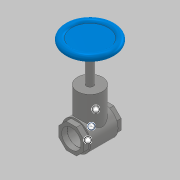
# Autodesk Inventor part: Manual Threaded Ball Valve DN40 S235
Saved by Autodesk Inventor 2017 (Build 210142000, 142)
## iProperties
Created: 2017-11-25
Part Number: Manual Threaded Ball Valve DN40 S235
Material: S235
Document SubType Name: Modeling
Designer: Demarec
Density: 7.85 g/cm^3
Appearance: Plate(1)
Catalog Web Link: http://www.pocketbrewery.com
Author: Demarec
Autodesk Inventor part; units mm, degrees
ref_plane "YZ Plane" through (0, 0, 0) normal (1, 0, 0) x (0, 1, 0)
ref_plane "XZ Plane" through (0, 0, 0) normal (0, 1, 0) x (-1, 0, 0)
ref_plane "XY Plane" through (0, 0, 0) normal (0, 0, 1) x (1, 0, 0)
sketch "Sketch3" plane through (0, 0, 0) normal (0, 1, 0) x (-1, 0, 0)
  line L0 (-11.3909, 27.5) -> (11.3909, 27.5)
  line L1 (11.3909, 27.5) -> (27.5, 11.3909)
  line L2 (27.5, 11.3909) -> (27.5, -11.3909)
  line L3 (27.5, -11.3909) -> (11.3909, -27.5)
  line L4 (11.3909, -27.5) -> (-11.3909, -27.5)
  line L5 (-11.3909, -27.5) -> (-27.5, -11.3909)
  line L6 (-27.5, -11.3909) -> (-27.5, 11.3909)
  line L7 (-27.5, 11.3909) -> (-11.3909, 27.5)
  circle A0 centre (0, 0) radius 29.7658
  circle A1 centre (0, 0) radius 27.5
  circle A2 centre (0, 0) radius 21
  circle A3 centre (0, 0) radius 31.7658
  line L8 (0, 0) -> (-27.5, 0)
  line L9 (-27.5, 0) -> (-27.5, 83)
  line L10 (-27.5, 83) -> (0, 83)
  line L11 (0, 83) -> (0, 0)
  line L12 (0, 83) -> (-7.5939, 83)
  line L13 (-7.5939, 83) -> (-7.5939, 166)
  line L14 (-7.5939, 166) -> (0, 166)
  line L15 (0, 166) -> (0, 83)
  line L16 (0, 166) -> (-47, 166)
  line L17 (-47, 166) -> (-47, 171)
  line L18 (-47, 171) -> (0, 171)
  line L19 (0, 171) -> (0, 166)
  circle A4 centre (-47, 168.5) radius 7.5939
  dimension "oSW" = 55
  dimension "oIntDia" = 42
  dimension "d16" = 2
  dimension "oWheelDia" = 94
  dimension "d51" = 5
  dimension "d52" = 15.1878
  dimension "oStemHeight" = 171
  dimension "d57" = 15.1878
  dimension "d58" = 22.7817
  constraints: 40 end point, 7 parallel, 4 centre point, 4 coincident, 4 horizontal, 3 perpendicular, 2 midpoint, 1 tangent, 20 other
  measures "oSW" distance between parallel lines of L6 L2
  measures "oIntDia" diameter of A2
  measures "oWheelDia" diameter of L17 L15
  measures "d51" distance of L18.end L14.end
  measures "d52" diameter of A4
  measures "oStemHeight" distance from line of A3.centre L18
  measures "d57" diameter of L13 L15
  measures "d58" distance of L0.start L0.end
revolve "Revolution1" add sketch "Sketch3" angle 360 about axis through (0, 0, 166) along (0, 0, -1) picked at (-6.365, 27.9172) picked at (-16.0373, 26.4927) picked at (-1.7883, 25.1572) picked at (-13.8245, 1.5576) contours A0 L11 L0 | L0 A1 L7 | L7 A0 | A0 L9 A3 L11 | L11 A2 L8 A1 | A1 L6 L7 | L11 L8 A2 | L9 L10 L11 A3 | L10 L13 L14 L15 | L14 L16 A4 L18 L19 | A4 L18 L17 L16 | L16 L17 L18 A4
extrude "Extrusion1" add sketch "Sketch3" along normal mid plane 82 separate body contours L0 A1 L7 | L0 L1 A1 | L11 A2 L8 A1 | A1 L8 A2 L11 | A1 L6 L7 | L1 L2 A1 | A1 L5 L6 | L2 L3 A1 | A1 L4 L5 | L3 L4 A1
extrude "Extrusion12" cut sketch "Sketch3" along normal through all both and the other way through all contours L11 L8 A2 | A2 L8 L11
extrude "Extrusion2" add sketch "Sketch3" along normal mid plane 60 contours A0 L11 L0 | L7 A0 | A0 L9 A3 L11 | L11 A0 L0 | L6 A0 | A0 L11 A3 L9 | A0 L1 | L5 A0 | A0 L2 | L4 A0 | A0 L3
sketch "Sketch10" plane through (0, 41, 0) normal (0, 1, 0) x (1, 0, 0)
  circle A0 centre (0, 0) radius 21 projected
  circle A1 centre (0, 0) radius 21.25
  dimension "d44" = 0.25
  constraints: 1 centre point
  measures "d44" radial gap between concentric circles of A0 A1
extrude "Extrusion11" cut sketch "Sketch10" against normal blind 12
mirror "Mirror1" about plane through (0, 0, 0) normal (0, 1, 0) of "Extrusion11"
equation "\"d52\" = 0.666667 * d58"
equation "\"d57\" = d52"
body "Solid1"
